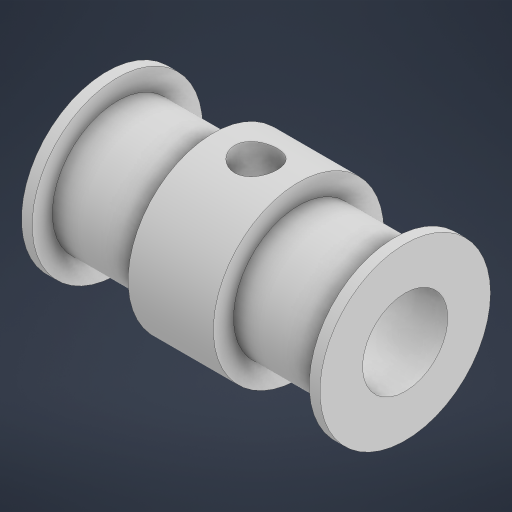
# Autodesk Inventor part: double_gt2
Saved by Autodesk Inventor 2024 (Build 280153000, 153)
## iProperties
Created: 2023-09-26
Part Number: double_gt2
Material: Типовые
Document SubType Name: Modeling
Designer: user
Density: 1 g/cm^3
Appearance: По умолчанию
Author: user
Autodesk Inventor part; units mm, degrees
ref_plane "YZ Plane" through (0, 0, 0) normal (1, 0, 0) x (0, 1, 0)
ref_plane "XY Plane" through (0, 0, 0) normal (0, 0, 1) x (1, 0, 0)
sketch "Эскиз1" plane through (0, 0, 0) normal (0, 0, 1) x (1, 0, 0)
  line L0 (10, 6.11) -> (10, 8)
  line L1 (10, 8) -> (18, 8)
  line L2 (18, 8) -> (18, 6.11)
  line L3 (18, 6.11) -> (27, 6.11)
  line L4 (27, 6.11) -> (27, 8)
  line L5 (27, 8) -> (28, 8)
  line L6 (28, 8) -> (28, 0)
  line L7 (0, 0) -> (0, 8)
  line L8 (0, 8) -> (1, 8)
  line L9 (1, 8) -> (1, 6.11)
  line L10 (1, 6.11) -> (10, 6.11)
  line L11 (0, 0) -> (28, 0)
  point P0 (22.5, 6.11)
  dimension "d0" = 6.11
  dimension "d1" = 8
  dimension "d2" = 28
  dimension "d4" = 9
  dimension "d5" = 8
  constraints: 24 end point, 8 perpendicular, 3 horizontal, 3 horizontal alignment, 2 collinear, 1 midpoint, 1 vertical
  measures "d0" vertical distance of L7.start L9.end
  measures "d1" distance of L7.end L7.start
  measures "d2" distance of L5.end L7.end
  measures "d4" distance of L1.end L4.end
  measures "d5" distance of L0.end L1.end
revolve "Вращение1" add sketch "Эскиз1" angle 360 about axis through (0, 0, 0) along (1, 0, 0)
sketch "Эскиз2" plane through (28, 0, 0) normal (1, 0, 0) x (0, 0, -1)
  circle A0 centre (0, 0) radius 4
  dimension "d7" = 8
  constraints: 1 centre point, 1 coincident
  measures "d7" diameter of A0
extrude "Выдавливание1" cut sketch "Эскиз2" against normal through all
ref_plane "РабПлоскость1" through (14, 8, 0) normal (0, 1, 0) x (-1, 0, 0)
sketch "Эскиз3" plane through (14, 8, 0) normal (0, 1, 0) x (-1, 0, 0)
  circle A0 centre (0, 0) radius 2
  line L0 (4, -8) -> (-4, -8) projected
  point P0 (14, 0)
  point P1 (0, -8)
  dimension "d10" = 4
  constraints: 1 centre point, 1 horizontal alignment, 1 midpoint, 1 vertical alignment
  measures "d10" diameter of A0
extrude "Выдавливание2" cut sketch "Эскиз3" against normal blind 6.5
pattern_circular "Круговой массив1" count 2 over 90 about axis through (14, 0, 0) along (1, 0, 0) of "Выдавливание2"
